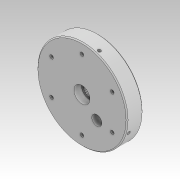
# Autodesk Inventor part: Wrist
Saved by Autodesk Inventor 2020 (Build 240168000, 168)
## iProperties
Created: 2021-03-19
Part Number: Wrist
Material: Generic
Document SubType Name: Modeling
Designer: DDeGo
Density: 1 g/cm^3
Appearance: Default
Author: DDeGo
Autodesk Inventor part; units mm, degrees
ref_plane "YZ Plane" through (0, 0, 0) normal (1, 0, 0) x (0, 1, 0)
ref_plane "XZ Plane" through (0, 0, 0) normal (0, 1, 0) x (-1, 0, 0)
ref_plane "XY Plane" through (0, 0, 0) normal (0, 0, 1) x (1, 0, 0)
sketch "Sketch1" plane through (0, 0, 0) normal (0, 0, 1) x (1, 0, 0)
  circle A0 centre (0, 0) radius 45
  circle A1 centre (0, 0) radius 5.65
  dimension "d0" = 11.3
  dimension "d1" = 90
  constraints: 2 centre point, 2 coincident
  measures "d0" diameter of A1
  measures "d1" diameter of A0
extrude "Extrusion1" add sketch "Sketch1" along normal blind 16
sketch "Sketch4" plane through (0, 0, 16) normal (0, 0, 1) x (1, 0, 0)
  circle A0 centre (0, 0) radius 5.65 construction
  circle A1 centre (-5.65, 0) radius 0.55
  line L0 (0, 0) -> (-5.65, 0) construction
  circle A2 centre (-5.3735, -1.7459) radius 0.55
  circle A3 centre (-4.5709, -3.321) radius 0.55
  circle A4 centre (-3.321, -4.5709) radius 0.55
  circle A5 centre (-1.7459, -5.3735) radius 0.55
  circle A6 centre (0, -5.65) radius 0.55
  circle A7 centre (1.7459, -5.3735) radius 0.55
  circle A8 centre (3.321, -4.5709) radius 0.55
  circle A9 centre (4.5709, -3.321) radius 0.55
  circle A10 centre (5.3735, -1.7459) radius 0.55
  circle A11 centre (5.65, 0) radius 0.55
  circle A12 centre (5.3735, 1.7459) radius 0.55
  circle A13 centre (4.5709, 3.321) radius 0.55
  circle A14 centre (3.321, 4.5709) radius 0.55
  circle A15 centre (1.7459, 5.3735) radius 0.55
  circle A16 centre (0, 5.65) radius 0.55
  circle A17 centre (-1.7459, 5.3735) radius 0.55
  circle A18 centre (-3.321, 4.5709) radius 0.55
  circle A19 centre (-4.5709, 3.321) radius 0.55
  circle A20 centre (-5.3735, 1.7459) radius 0.55
  dimension "d15" = 1.1
  dimension "d18" = 360
  constraints: 20 centre point, 2 end point, 1 horizontal, 1 horizontal alignment, 42 other
  measures "d15" diameter of A1
extrude "Extrusion5" cut sketch "Sketch4" against normal through all
sketch "Sketch5" plane through (0, 0, 16) normal (0, 0, 1) x (1, 0, 0)
  circle A0 centre (0, 0) radius 8
  dimension "d22" = 16
  constraints: 1 centre point, 1 coincident
  measures "d22" diameter of A0
extrude "Extrusion6" cut sketch "Sketch5" against normal blind 7.5
sketch "Sketch6" plane through (0, 0, 0) normal (0, 0, -1) x (-1, 0, 0)
  line L0 (0, 0) -> (0, 35) construction
  circle A0 centre (0, 35) radius 1.75
  circle A1 centre (-30.3109, 17.5) radius 1.75
  circle A2 centre (-30.3109, -17.5) radius 1.75
  circle A3 centre (0, -35) radius 1.75
  circle A4 centre (30.3109, -17.5) radius 1.75
  circle A5 centre (30.3109, 17.5) radius 1.75
  dimension "d25" = 3.5
  dimension "d26" = 35
  dimension "d29" = 360
  constraints: 6 centre point, 6 coincident, 2 end point, 1 vertical, 19 other
  measures "d25" diameter of A0
  measures "d26" distance of L0.start L0.end
extrude "Extrusion7" cut sketch "Sketch6" against normal through all
sketch "Sketch7" plane through (0, 0, 0) normal (0, 0, -1) x (-1, 0, 0)
  line L0 (-2.8, 32.2) -> (2.8, 32.2)
  line L1 (2.8, 32.2) -> (2.8, 37.8)
  line L2 (2.8, 37.8) -> (-2.8, 37.8)
  line L3 (-2.8, 37.8) -> (-2.8, 32.2)
  circle A0 centre (0, 35) radius 1.75 construction
  line L4 (-2.8, 32.2) -> (2.8, 37.8) construction
  line L5 (2.8, 32.2) -> (-2.8, 37.8) construction
  point P0 (0, 0)
  dimension "d33" = 5.6
  constraints: 12 end point, 2 midpoint, 2 parallel, 2 perpendicular, 1 horizontal
  measures "d33" distance of L1.end L2.end
extrude "Extrusion8" cut sketch "Sketch7" against normal blind 3
sketch "Sketch8" plane through (0, 0, 3) normal (0, 0, -1) x (-1, 0, 0)
  line L0 (-2.8, 37.8) -> (2.8, 37.8) projected
  line L1 (-2.8, 37.8) -> (-1.75, 37.8)
  line L2 (-1.75, 37.8) -> (-1.75, 32.2)
  line L3 (-1.75, 32.2) -> (-2.8, 32.2)
  line L4 (-2.8, 32.2) -> (-2.8, 37.8)
  line L5 (2.8, 32.2) -> (-2.8, 32.2) projected
  line L6 (2.8, 37.8) -> (1.75, 37.8)
  line L7 (1.75, 37.8) -> (1.75, 32.2)
  line L8 (1.75, 32.2) -> (2.8, 32.2)
  line L9 (2.8, 32.2) -> (2.8, 37.8)
  circle A0 centre (0, 35) radius 1.75 projected
  point P0 (0, 0)
  point P1 (-1.75, 35)
  point P2 (1.75, 35)
  constraints: 16 end point, 4 parallel, 2 horizontal, 2 perpendicular, 2 point on line, 2 tangent
extrude "Extrusion9" cut sketch "Sketch8" against normal blind 0.2 contours L0 L7 A0 L2 | A0 L7 L5 L2
sketch "Sketch9" plane through (0, 0, 3.2) normal (0, 0, -1) x (-1, 0, 0)
  line L0 (-1.75, 37.8) -> (1.75, 37.8) projected
  line L1 (1.75, 37.8) -> (1.75, 32.2) projected
  line L2 (-1.75, 37.8) -> (1.75, 37.8)
  line L3 (1.75, 37.8) -> (1.75, 36.75)
  line L4 (1.75, 36.75) -> (-1.75, 36.75)
  line L5 (-1.75, 36.75) -> (-1.75, 37.8)
  line L6 (-1.75, 32.2) -> (-1.75, 37.8) projected
  line L7 (1.75, 32.2) -> (-1.75, 32.2)
  line L8 (-1.75, 32.2) -> (-1.75, 33.25)
  line L9 (-1.75, 33.25) -> (1.75, 33.25)
  line L10 (1.75, 33.25) -> (1.75, 32.2)
  arc A0 (1.75, 35) -> (-1.75, 35) centre (0, 35) ccw projected
  arc A1 (-1.75, 35) -> (1.75, 35) centre (0, 35) ccw projected
  point P0 (0, 0)
  point P1 (0, 33.25)
  point P2 (0, 36.75)
  constraints: 16 end point, 4 parallel, 2 horizontal, 2 perpendicular, 2 point on line, 2 tangent
extrude "Extrusion10" cut sketch "Sketch9" against normal blind 0.2 contours L4 A0 L6 | L1 A0 L4 | A1 L9 L6 | L1 L9 A1
pattern_circular "Circular Pattern1" count 6 over 360 about axis through (0, 0, 16) along (0, 0, -1) of "Extrusion8", "Extrusion9", "Extrusion10"
sketch "Sketch10" plane through (0, 0, 0) normal (0, 0, -1) x (-1, 0, 0)
  arc A0 (0, -25) -> (-25, 0) centre (0, 0) ccw construction
  arc A1 (0, -29) -> (-29, 0) centre (0, 0) ccw
  arc A2 (0, -21) -> (-21, 0) centre (0, 0) ccw
  arc A3 (0, -21) -> (0, -29) centre (0, -25) ccw
  arc A4 (-29, 0) -> (-21, 0) centre (-25, 0) ccw
  line L0 (0, -25) -> (0, 0) construction
  line L1 (0, 0) -> (-25, 0) construction
  dimension "d43" = 25
  dimension "d44" = 4
  constraints: 10 point on circle, 5 centre point, 4 end point, 4 tangent, 1 coincident, 1 perpendicular, 1 vertical
  measures "d43" radius of A0
  measures "d44" radius of A3
extrude "Extrusion11" cut sketch "Sketch10" against normal blind 7
sketch "Sketch11" plane through (0, 0, 7) normal (0, 0, -1) x (-1, 0, 0)
  arc A0 (0, -29) -> (-29, 0) centre (0, 0) ccw projected
  circle A1 centre (0, 0) radius 29
  circle A2 centre (0, 0) radius 21
  point P0 (-21, 0)
  point P1 (0, -29)
  constraints: 2 coincident, 1 horizontal alignment, 5 other
extrude "Extrusion12" cut sketch "Sketch11" along normal blind 4
sketch "Sketch12" plane through (0, 0, 16) normal (0, 0, 1) x (1, 0, 0)
  arc A0 (0, -21) -> (21, 0) centre (0, 0) ccw construction
  circle A1 centre (14.8492, -14.8492) radius 5
  dimension "d49" = 10
  constraints: 2 point on circle, 1 centre point
  measures "d49" diameter of A1
extrude "Extrusion13" cut sketch "Sketch12" against normal up to surface (9 mm away)
ref_plane "Work Plane1" through (0, 0, 12.25) normal (0, 0, 1) x (1, 0, 0)
sketch "Sketch13" plane through (0, 0, 12.25) normal (0, 0, 1) x (1, 0, 0)
  line L0 (0, 0) -> (47.6858, -15.0353)
  line L1 (0, 0) -> (15.0353, 47.6858)
  line L2 (0, 0) -> (0, 55.5224) construction
  dimension "d58" = 90
  dimension "d59" = 50
  dimension "d60" = 17.5
  constraints: 6 end point, 2 coincident, 1 perpendicular, 1 vertical
  measures "d58" angle of L0 L1
  measures "d59" distance of L0.start L1.end
  measures "d60" angle of L1 L2
ref_plane "Work Plane2" through (47.6858, -15.0353, 12.25) normal (0.953717, -0.3007058, 0) x (0.3007058, 0.953717, 0)
ref_plane "Work Plane3" through (15.0353, 47.6858, 12.25) normal (0.3007058, 0.953717, 0) x (-0.953717, 0.3007058, 0)
sketch "Sketch14" plane through (15.0353, 47.6858, 12.25) normal (0.3007058, 0.953717, 0) x (-0.953717, 0.3007058, 0)
  circle A0 centre (0, 0) radius 1.5
  point P0 (0, -12.25)
  point P1 (0, 0)
  dimension "d52" = 3
  constraints: 1 centre point, 1 coincident
  measures "d52" diameter of A0
extrude "Extrusion14" cut sketch "Sketch14" against normal up to surface (50 mm away)
sketch "Sketch15" plane through (47.6858, -15.0353, 12.25) normal (0.953717, -0.3007058, 0) x (0.3007058, 0.953717, 0)
  circle A0 centre (0, 0) radius 1.5
  point P0 (0, -12.25)
  point P1 (0, 0)
  dimension "d55" = 3
  constraints: 1 centre point, 1 coincident
  measures "d55" diameter of A0
extrude "Extrusion15" cut sketch "Sketch15" against normal up to surface (50 mm away)
chamfer "Chamfer1" distance 1 angle 45 2 edges at (-45, 0, 0) (-45, 0, 16)
body "Solid1"
